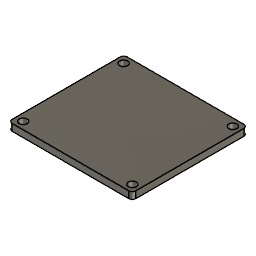
Plaid case (Autodesk Fusion 360 design; units mm, degrees)
part number: 2025-12-06-16-52-57-663
Autodesk Fusion 360 part; units mm, degrees
sketch "Sketch1" plane through (0, 0, 0) normal (0, 0, 1) x (1, 0, 0)
  line L0 (0, 0) -> (72, 0)
  line L1 (72, 0) -> (72, 67)
  line L2 (72, 67) -> (0, 67)
  line L3 (0, 67) -> (0, 0)
  circle A0 centre (4.25, 62.71) radius 1.7
  circle A1 centre (67.75, 62.71) radius 1.7
  circle A2 centre (4.25, 4.29) radius 1.7
  circle A3 centre (67.75, 4.29) radius 1.7
  circle A4 centre (4.25, 62.71) radius 2.35
  circle A5 centre (67.75, 62.71) radius 2.35
  circle A6 centre (67.75, 4.29) radius 2.35
  circle A7 centre (4.25, 4.29) radius 2.35
  dimension "d1" = 67
  dimension "d2" = 72
  dimension "d3" = 3.4
  dimension "d4" = 3.4
  dimension "d5" = 3.4
  dimension "d6" = 3.4
  dimension "d7" = 4.25
  dimension "d8" = 4.29
  dimension "d9" = 4.25
  dimension "d10" = 4.29
  dimension "d11" = 4.29
  dimension "d12" = 4.25
  dimension "d13" = 4.25
  dimension "d14" = 4.29
  dimension "d15" = 4.7
  dimension "d16" = 4.7
  dimension "d17" = 4.7
  dimension "d18" = 4.7
  constraint horizontal L0
  constraint vertical L1
  constraint horizontal L2
  constraint vertical L3
  constraint coincident L0.start L3.end
  constraint concentric A0 A4
  constraint concentric A1 A5
  constraint concentric A3 A6
  constraint concentric A2 A7
  measures "d1" distance of L0.start L2.end
  measures "d2" distance of L1.end L2.end
  measures "d3" diameter of A0
  measures "d4" diameter of A1
  measures "d5" diameter of A2
  measures "d6" diameter of A3
  measures "d7" distance of L3 A2.centre
  measures "d8" distance of L0 A2.centre
  measures "d9" distance of L1 A3.centre
  measures "d10" distance of L0 A3.centre
  measures "d11" distance of L2 A1.centre
  measures "d12" distance of L1 A1.centre
  measures "d13" distance of L3 A0.centre
  measures "d14" distance of L2 A0.centre
  measures "d15" diameter of A4
  measures "d16" diameter of A5
  measures "d17" diameter of A6
  measures "d18" diameter of A7
extrude "Extrude1" add sketch "Sketch1" along normal blind 4 contours L0 L1 L2 L3
fillet "Fillet1" radius 2 1 edges at (0, 0, 2)
fillet "Fillet2" radius 2 1 edges at (72, 0, 2)
fillet "Fillet3" radius 2 1 edges at (72, 67, 2)
fillet "Fillet4" radius 2 1 edges at (0, 67, 2)
sketch "Sketch2" plane through (0, 0, 0) normal (0, 0, 1) x (1, 0, 0)
sketch "Sketch3" plane through (0, 0, 0) normal (0, 0, 1) x (1, 0, 0)
  line L0 (60, 63) -> (51, 63) construction
  line L1 (51, 63) -> (51, 65) construction
  line L2 (51, 65) -> (60, 65) construction
  line L3 (60, 65) -> (60, 63) construction
  dimension "d29" = 1.5
  dimension "d30" = 0
  text T0 "IBN 5100" font "Arial" height 1.5 align left top in box 9 x 2 at (60, 63) x (-1, 0) y (0, 1) spacing 1
extrude "Extrude2" add sketch "Sketch3" against normal blind 0.2 text T0
equation "d30 = 'IBN 5100'"
